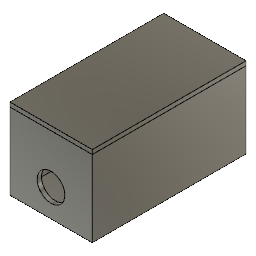
pedal-input (Autodesk Fusion 360 design; units mm, degrees)
Autodesk Fusion 360 part; units mm, degrees
sketch "Sketch1" plane through (0, 0, 0) normal (0, 1, 0) x (1, 0, 0) in component "Case"
  circle A0 centre (0, 0) radius 6.15
  dimension "d9" = 12.3
  constraint coincident A0.centre origin
  measures "d9" diameter of A0
extrude "Extrude2" add sketch "Sketch1" along normal blind 40.4 makes body 1 in component "Case"
sketch "Sketch2" plane through (0, 0, 0) normal (0, -1, 0) x (1, 0, 0) in component "Case"
  circle A0 centre (0, 0) radius 6.15
  circle A1 centre (0, 0) radius 4.85
  dimension "d12" = 9.7
  constraint coincident A0.centre A1.centre
  measures "d12" diameter of A1
extrude "Extrude3" add sketch "Sketch2" along normal blind 2.7 contours A1 bodies 1 in component "Case"
sketch "Sketch3" plane through (0, -2.7, 0) normal (0, -1, 0) x (1, 0, 0) in component "Case"
  circle A0 centre (0, 0) radius 4.85
  circle A1 centre (0, 0) radius 3.3
  dimension "d15" = 6.6
  constraint coincident A0.centre A1.centre
  measures "d15" diameter of A1
extrude "Extrude4" cut sketch "Sketch3" against normal up to surface (42.1 mm away) contours A1 bodies 1 in component "Case"
sketch "Sketch4" plane through (0, 40.4, 0) normal (0, 1, 0) x (-1, 0, 0) in component "Case"
  circle A0 centre (0, 0) radius 6.15
  line L0 (0, 0) -> (2.1, 0)
  line L1 (0, 0) -> (-2.1, 0)
  line L2 (-1.95, 1.525) -> (-2.25, 1.525)
  line L3 (-2.25, 1.525) -> (-2.25, -1.525)
  line L4 (-2.25, -1.525) -> (-1.95, -1.525)
  line L5 (-1.95, -1.525) -> (-1.95, 1.525)
  line L6 (-1.95, 1.525) -> (-2.25, -1.525) construction
  line L7 (-2.25, 1.525) -> (-1.95, -1.525) construction
  line L8 (2.25, 1.525) -> (1.95, 1.525)
  line L9 (1.95, 1.525) -> (1.95, -1.525)
  line L10 (1.95, -1.525) -> (2.25, -1.525)
  line L11 (2.25, -1.525) -> (2.25, 1.525)
  line L12 (2.25, 1.525) -> (1.95, -1.525) construction
  line L13 (1.95, 1.525) -> (2.25, -1.525) construction
  point P0 (-2.1, 0)
  point P1 (2.1, 0)
  dimension "d19" = 2.1
  dimension "d20" = 2.1
  dimension "d21" = 0.3
  dimension "d22" = 3.05
  dimension "d25" = 0.3
  dimension "d26" = 3.05
  constraint coincident A0.centre L0.start
  constraint horizontal L0
  constraint parallel L0 L1
  constraint horizontal L2
  constraint perpendicular L2 L3
  constraint parallel L2 L4
  constraint parallel L3 L5
  constraint coincident L6 P0
  constraint coincident L7 P0
  constraint coincident P0 L1.end
  constraint horizontal L8
  constraint perpendicular L8 L9
  constraint parallel L8 L10
  constraint parallel L9 L11
  constraint coincident L12 P1
  constraint coincident L13 P1
  constraint coincident P1 L0.end
  measures "d19" distance of A0.centre P1
  measures "d20" distance of A0.centre P0
  measures "d21" distance of L3.end L4.end
  measures "d22" distance of L2.end L3.end
  measures "d25" distance of L9.end L10.end
  measures "d26" distance of L8.end L9.end
extrude "Extrude5" add sketch "Sketch4" along normal blind 4 contours L2 L3 L4 L5 | L8 L9 L10 L11 bodies 1 in component "Case"
sketch "Sketch5" plane through (0, 0, 0) normal (0, -1, 0) x (1, 0, 0) in component "Case"
  circle A0 centre (0, 0) radius 4.85
  circle A1 centre (0, 0) radius 6.15
  line L0 (12.95, 8.15) -> (-12.95, 8.15)
  line L1 (-12.95, 8.15) -> (-12.95, -8.15)
  line L2 (-12.95, -8.15) -> (12.95, -8.15)
  line L3 (12.95, -8.15) -> (12.95, 8.15)
  line L4 (12.95, 8.15) -> (-12.95, -8.15) construction
  line L5 (-12.95, 8.15) -> (12.95, -8.15) construction
  line L6 (-12.95, 8.15) -> (12.95, 8.15)
  line L7 (12.95, 8.15) -> (12.95, 17.15)
  line L8 (12.95, 17.15) -> (-12.95, 17.15)
  line L9 (-12.95, 17.15) -> (-12.95, 8.15)
  line L10 (14.45, 6.65) -> (14.45, 18.65)
  line L11 (14.45, 18.65) -> (-14.45, 18.65)
  line L12 (-14.45, 18.65) -> (-14.45, 6.65)
  line L13 (-14.45, 6.65) -> (14.45, 6.65)
  line L14 (-14.45, 9.65) -> (-14.45, -9.65)
  line L15 (-14.45, -9.65) -> (14.45, -9.65)
  line L16 (14.45, -9.65) -> (14.45, 9.65)
  line L17 (14.45, 9.65) -> (-14.45, 9.65)
  dimension "d35" = 25.9
  dimension "d36" = 16.3
  dimension "d37" = 25.9
  dimension "d38" = 9
  dimension "d41" = 1.5
  dimension "d42" = 1.5
  constraint horizontal L0
  constraint perpendicular L0 L1
  constraint parallel L0 L2
  constraint parallel L1 L3
  constraint coincident L4 A0.centre
  constraint coincident L5 A0.centre
  constraint coincident A0.centre A1.centre
  constraint horizontal L6
  constraint vertical L7
  constraint horizontal L8
  constraint vertical L9
  measures "d35" distance of L1.end L2.end
  measures "d36" distance of L0.end L1.end
  measures "d37" distance of L0.end L0.start
  measures "d38" distance of L0.end L8.end
extrude "Extrude6" add sketch "Sketch5" along normal blind 1.5 separate body contours A1 | L0 L1 L3 L6 L13 | L3 L7 L10 L13 L16 L17 | L0 L6 L7 L9 L17 | L1 L9 L12 L13 L14 L17 | L1 L2 L3 L13 L14 L15 L16 | L1 L2 L3 L13 | L7 L8 L9 L17 | L7 L8 L9 L10 L11 L12 L17 makes body 2 in component "Case"
sketch "Sketch6" plane through (0, 0, 0) normal (0, 1, 0) x (-1, 0, 0) in component "Case"
  line L0 (-14.45, 18.65) -> (-14.45, -9.65)
  line L1 (-14.45, -9.65) -> (14.45, -9.65)
  line L2 (14.45, -9.65) -> (14.45, 18.65)
  line L3 (14.45, 18.65) -> (-14.45, 18.65)
  line L4 (-12.95, -8.15) -> (12.95, -8.15)
  line L5 (12.95, -8.15) -> (12.95, 17.15)
  line L6 (12.95, 17.15) -> (-12.95, 17.15)
  line L7 (-12.95, 17.15) -> (-12.95, -8.15)
  circle A0 centre (0, 0) radius 4.85
extrude "Extrude7" add sketch "Sketch6" along normal blind 51.4 contours L0 L1 L2 L3 bodies 1 2 in component "Case"
sketch "Sketch7" plane through (0, 0, 17.15) normal (0, 0, -1) x (1, 0, 0) in component "Case"
  line L0 (12.95, 0) -> (-12.95, 0)
  line L1 (-12.95, 0) -> (-12.95, -51.4)
  line L2 (-12.95, -51.4) -> (12.95, -51.4)
  line L3 (12.95, -51.4) -> (12.95, 0)
  line L4 (12.95, 0) -> (-12.95, -51.4) construction
  line L5 (12.95, -51.4) -> (-12.95, 0) construction
  line L6 (-5, -30.5) -> (5, -30.5)
  line L7 (5, -30.5) -> (5, -45.5)
  line L8 (5, -45.5) -> (-5, -45.5)
  line L9 (-5, -45.5) -> (-5, -30.5)
  line L10 (-5, -30.5) -> (5, -45.5) construction
  line L11 (5, -30.5) -> (-5, -45.5) construction
  point P0 (0, -38)
  dimension "d54" = 10
  dimension "d55" = 15
  constraint coincident L0.start L3.end
  constraint coincident L1.end L2.start
  constraint coincident L2.end L3.start
  constraint coincident L0.end L1.start
  constraint horizontal L6
  constraint perpendicular L6 L7
  constraint parallel L6 L8
  constraint parallel L7 L9
  constraint coincident L10 P0
  constraint coincident L11 P0
  measures "d54" distance of L7.end L8.end
  measures "d55" distance of L6.end L7.end
extrude "Extrude9" add sketch "Sketch7" along normal blind 4 separate body contours L6 L7 L8 L9 makes body 3 in component "Case"
sketch "Sketch8" plane through (0, 0, 13.15) normal (0, 0, -1) x (1, 0, 0) in component "Case"
  line L0 (-5, -45.5) -> (5, -45.5)
  line L1 (5, -45.5) -> (5, -30.5)
  line L2 (5, -30.5) -> (-5, -30.5)
  line L3 (-5, -30.5) -> (-5, -45.5)
  line L4 (12.95, 0) -> (-12.95, 0)
  line L5 (-12.95, 0) -> (-12.95, -51.4)
  line L6 (-12.95, -51.4) -> (12.95, -51.4)
  line L7 (12.95, -51.4) -> (12.95, 0)
  line L8 (12.95, -51.4) -> (-12.95, -51.4)
  line L9 (-12.95, -51.4) -> (-12.95, -17.05)
  line L10 (-12.95, -17.05) -> (12.95, -17.05)
  line L11 (12.95, -17.05) -> (12.95, -51.4)
  dimension "d58" = 25.9
  dimension "d59" = 34.35
  constraint horizontal L8
  constraint vertical L9
  constraint horizontal L10
  constraint vertical L11
  constraint coincident L6.end L7.start
  measures "d58" distance of L6.end L5.end
  measures "d59" distance of L6.end L10.end
extrude "Extrude10" add sketch "Sketch8" along normal blind 1 contours L0 L1 L2 L3 | L5 L6 L7 L8 L9 L10 L11 bodies 3 in component "Case"
sketch "Sketch9" plane through (0, 0, 12.15) normal (0, 0, -1) x (1, 0, 0) in component "Case"
  line L0 (12.95, -17.05) -> (-12.95, -17.05)
  line L1 (-12.95, -17.05) -> (-12.95, -51.4)
  line L2 (-12.95, -51.4) -> (12.95, -51.4)
  line L3 (12.95, -51.4) -> (12.95, -17.05)
  line L4 (4.15, -46.5756) -> (-4.15, -46.5756)
  line L5 (-4.15, -46.5756) -> (-4.15, -56.2244)
  line L6 (-4.15, -56.2244) -> (4.15, -56.2244)
  line L7 (4.15, -56.2244) -> (4.15, -46.5756)
  line L8 (4.15, -46.5756) -> (-4.15, -56.2244) construction
  line L9 (-4.15, -46.5756) -> (4.15, -56.2244) construction
  point P0 (0, -51.4)
  dimension "d65" = 8.3
  constraint horizontal L4
  constraint perpendicular L4 L5
  constraint parallel L4 L6
  constraint parallel L5 L7
  constraint coincident L8 P0
  constraint coincident L9 P0
  constraint midpoint L2 P0
  measures "d65" distance of L5.end L6.end
extrude "Extrude11" add sketch "Sketch9" along normal blind 2.9 contours L2 L4 L5 L7 bodies 3 in component "Case"
sketch "Sketch10" plane through (0, 0, -8.15) normal (0, 0, 1) x (-1, 0, 0) in component "Case"
  line L0 (12.95, 0) -> (-12.95, 0)
  line L1 (-12.95, 0) -> (-12.95, -51.4)
  line L2 (-12.95, -51.4) -> (12.95, -51.4)
  line L3 (12.95, -51.4) -> (12.95, 0)
  line L4 (-12.95, 0) -> (-12.95, -41.9) construction
  line L5 (-12.95, -41.9) -> (12.95, -41.9)
  line L6 (12.95, -41.9) -> (12.95, -35.9)
  line L7 (12.95, -35.9) -> (-12.95, -35.9)
  line L8 (-12.95, -35.9) -> (-12.95, -41.9)
  dimension "d81" = 41.9
  dimension "d82" = 25.9
  dimension "d83" = 6
  constraint coincident L0.end L1.start
  constraint perpendicular L0 L4
  constraint horizontal L5
  constraint vertical L6
  constraint horizontal L7
  constraint vertical L8
  measures "d81" distance of L0.end L4.end
  measures "d82" distance of L4.end L5.end
  measures "d83" distance of L4.end L7.end
extrude "Extrude16" add sketch "Sketch10" along normal blind 6.625 contours L1 L3 L5 L6 L7 L8 bodies 2 in component "Case"
sketch "Sketch11" plane through (0, 35.9, 0) normal (0, -1, 0) x (1, 0, 0) in component "Case"
  line L0 (-12.95, -8.15) -> (12.95, -8.15)
  line L1 (12.95, -8.15) -> (12.95, -1.525)
  line L2 (-12.95, -1.525) -> (-12.95, -8.15)
  line L3 (12.95, -1.525) -> (-12.95, -1.525)
  circle A0 centre (0, 0) radius 6.15
extrude "Extrude17" cut sketch "Sketch11" against normal blind 4.5 contours L3 A0 picked at (-0.9187, -4.796) bodies 2 in component "Case"
sketch "Sketch12" plane through (12.95, 0, 0) normal (-1, 0, 0) x (0, -1, 0) in component "Case"
  line L0 (-41.9, -8.15) -> (-41.9, -1.525)
  line L1 (-41.9, -1.525) -> (-35.9, -1.525)
  line L2 (0, -8.15) -> (0, 17.15)
  line L3 (0, 17.15) -> (-51.4, 17.15)
  line L4 (-51.4, 17.15) -> (-51.4, -8.15)
  line L5 (-35.9, -8.15) -> (0, -8.15)
  line L6 (-51.4, 12.15) -> (-17.05, 12.15)
  line L7 (-25.6375, 10.65) -> (-42.8125, 10.65)
  line L8 (-42.8125, 10.65) -> (-42.8125, 13.65)
  line L9 (-42.8125, 13.65) -> (-25.6375, 13.65)
  line L10 (-25.6375, 13.65) -> (-25.6375, 10.65)
  line L11 (-25.6375, 10.65) -> (-42.8125, 13.65) construction
  line L12 (-42.8125, 10.65) -> (-25.6375, 13.65) construction
  line L13 (-35.9, -1.525) -> (-35.9, -8.15)
  line L14 (-17.05, 12.15) -> (-15.55, 12.15)
  line L15 (-15.55, 12.15) -> (-15.55, 13.65)
  line L16 (-15.55, 13.65) -> (-17.05, 13.65)
  line L17 (-17.05, 13.65) -> (-17.05, 12.15)
  line L18 (-51.4, -8.15) -> (-41.9, -8.15)
  point P0 (-34.225, 12.15)
  dimension "d94" = 17.175
  dimension "d95" = 3
  dimension "d106" = 1.5
  dimension "d107" = 1.5
  constraint horizontal L7
  constraint perpendicular L7 L8
  constraint parallel L7 L9
  constraint parallel L8 L10
  constraint coincident L11 P0
  constraint coincident L12 P0
  constraint midpoint L6 P0
  constraint horizontal L14
  constraint vertical L15
  constraint horizontal L16
  constraint vertical L17
  constraint coincident L6.end L14.start
  measures "d94" distance of L8.end L9.end
  measures "d95" distance of L7.end L8.end
  measures "d106" distance of L6.end L14.end
  measures "d107" distance of L6.end L16.end
extrude "Extrude22" add sketch "Sketch12" along normal blind 3.7 contours L14 L15 L16 L17 bodies 2 in component "Case"
extrude "Extrude20" add sketch "Sketch12" along normal blind 2.59 contours L6 L7 L8 L10 bodies 2 in component "Case"
sketch "Sketch13" plane through (-12.95, 0, 0) normal (1, 0, 0) x (0, 1, 0) in component "Case"
  line L0 (41.9, -1.525) -> (41.9, -8.15)
  line L1 (41.9, -8.15) -> (51.4, -8.15)
  line L2 (51.4, -8.15) -> (51.4, 17.15)
  line L3 (51.4, 17.15) -> (0, 17.15)
  line L4 (0, 17.15) -> (0, -8.15)
  line L5 (35.9, -1.525) -> (41.9, -1.525)
  line L6 (17.05, 12.15) -> (51.4, 12.15)
  line L7 (42.8125, 10.65) -> (25.6375, 10.65)
  line L8 (25.6375, 10.65) -> (25.6375, 13.65)
  line L9 (25.6375, 13.65) -> (42.8125, 13.65)
  line L10 (42.8125, 13.65) -> (42.8125, 10.65)
  line L11 (42.8125, 10.65) -> (25.6375, 13.65) construction
  line L12 (25.6375, 10.65) -> (42.8125, 13.65) construction
  line L13 (0, -8.15) -> (35.9, -8.15)
  line L14 (35.9, -8.15) -> (35.9, -1.525)
  line L15 (17.05, 12.15) -> (15.55, 12.15)
  line L16 (15.55, 12.15) -> (15.55, 13.65)
  line L17 (15.55, 13.65) -> (17.05, 13.65)
  line L18 (17.05, 13.65) -> (17.05, 12.15)
  point P0 (34.225, 12.15)
  dimension "d98" = 17.175
  dimension "d99" = 3
  dimension "d114" = 1.5
  dimension "d115" = 1.5
  constraint horizontal L7
  constraint perpendicular L7 L8
  constraint parallel L7 L9
  constraint parallel L8 L10
  constraint coincident L11 P0
  constraint coincident L12 P0
  constraint midpoint L6 P0
  constraint horizontal L15
  constraint vertical L16
  constraint horizontal L17
  constraint vertical L18
  constraint coincident L6.start L15.start
  measures "d98" distance of L8.end L9.end
  measures "d99" distance of L7.end L8.end
  measures "d114" distance of L6.start L15.end
  measures "d115" distance of L6.start L17.end
extrude "Extrude23" add sketch "Sketch13" along normal blind 3.7 contours L15 L16 L17 L18 bodies 2 in component "Case"
extrude "Extrude21" add sketch "Sketch13" along normal blind 2.59 contours L6 L7 L8 L10 bodies 2 in component "Case"
sketch "Sketch14" plane through (0, 51.4, 0) normal (0, 1, 0) x (-1, 0, 0) in component "Case"
  line L0 (-12.95, -8.15) -> (-12.95, 17.15)
  line L1 (-12.95, 17.15) -> (12.95, 17.15)
  line L2 (12.95, -8.15) -> (-12.95, -8.15)
  line L3 (14.45, 18.65) -> (-14.45, 18.65)
  line L4 (-14.45, 18.65) -> (-14.45, -9.65)
  line L5 (-14.45, -9.65) -> (14.45, -9.65)
  line L6 (14.45, -9.65) -> (14.45, 18.65)
  line L7 (12.95, 17.15) -> (12.95, -8.15)
extrude "Extrude18" add sketch "Sketch14" along normal blind 1 contours L0 L1 L2 L7 | L3 L4 L5 L6 bodies 2 in component "Case"
sketch "Sketch15" plane through (0, 51.4, 0) normal (0, 1, 0) x (-1, 0, 0) in component "Case"
  line L0 (12.95, 13.15) -> (-12.95, 13.15)
  line L1 (-12.95, 13.15) -> (-12.95, 12.15)
  line L2 (-12.95, 12.15) -> (-4.15, 12.15)
  line L3 (-4.15, 12.15) -> (-4.15, 9.25)
  line L4 (-4.15, 9.25) -> (4.15, 9.25)
  line L5 (4.15, 9.25) -> (4.15, 12.15)
  line L6 (4.15, 12.15) -> (12.95, 12.15)
  line L7 (12.95, 12.15) -> (12.95, 13.15)
  line L8 (-4.15, 12.15) -> (4.15, 12.15)
  dimension "d91" = 8.3
  constraint coincident L2.end L3.start
  constraint coincident L5.end L6.start
  measures "d91" distance of L2.end L5.end
extrude "Extrude19" cut sketch "Sketch15" along normal blind 1 contours L3 L4 L5 L8 bodies 2 in component "Case"
fillet "Fillet2" [suppressed] in component "Case"
split "Split1" by plane through (-12.95, 0, 17.15) normal (0, 0, -1) bodies 2 makes body 4 at (4.8167, 16.4667, -9.65) in component "Case"
component "Case" placed x (1, 0, 0) y (0, 1, 0) z (0, 0, 1) at (0, 0, 0)
hidden bodies 1 3
equation "JackLength = 39.4 mm + 1 mm" comment "Length of the jack without contacts or lip"
equation "JackDiameter = 11.3 mm + 1 mm" comment "Diameter of the jack"
equation "JackLipLength = 2.7 mm" comment "Length/height of the lip in the front of the jack"
equation "JackLipDiameter = 8.7 mm + 1 mm" comment "Diameter of the lip in the front of the jack"
equation "d9 = JackDiameter"
equation "d10 = JackLength"
equation "d12 = JackLipDiameter"
equation "d13 = JackLipLength"
equation "JackContactSpacing = 4.2 mm" comment "Space between the two contacts on the back of the jack"
equation "d19 = JackContactSpacing / 2"
equation "d20 = JackContactSpacing / 2"
equation "d21 = JackContactThickness"
equation "d22 = JackContactHeight"
equation "JackContactThickness = 0.3 mm" comment "Thickness of the contacts on the back of the jack"
equation "JackContactHeight = 2.8 mm + 0.25 mm" comment "Height of the contacts on the back of the jack"
equation "d25 = JackContactThickness"
equation "d26 = JackContactHeight"
equation "JackContactLength = 4 mm" comment "Length of the contact on the back of the jack"
equation "d28 = JackContactLength"
equation "ChipWidth = 25.4 mm + 0.5 mm" comment "Width of the Chip"
equation "ChipLength = 34.1 mm + 0.25 mm" comment "Length of the Chip"
equation "ChipThickness = 1 mm" comment "Chip PCB thickness"
equation "ChipBellyThickness = 3 mm + 1 mm" comment "Thickness/height of the \"belly\" of the chip"
equation "JackSpacing = 2 mm" comment "Space above and below jack"
equation "d35 = ChipWidth"
equation "d36 = 2 * ( JackDiameter / 2 + JackSpacing )"
equation "d37 = ChipWidth"
equation "d38 = ChipSpacing * 2 + ChipBellyThickness + ChipThickness"
equation "ChipSpacing = 2 mm" comment "Spacing under chip"
equation "WallThickness = 1.5 mm" comment "Thickness of all walls"
equation "d41 = WallThickness"
equation "d42 = WallThickness"
equation "d43 = WallThickness"
equation "d45 = -WallThickness"
equation "JackBackSpacing = 5 mm" comment "Spacing behind the contacts of the jack"
equation "d47 = JackLength + JackContactLength + ChipSpacing + JackBackSpacing"
equation "ChipUSBThickness = 2.4 mm + 0.5 mm" comment "Thickness/height of the USB connector"
equation "d56 = ChipBellyThickness"
equation "d58 = ChipWidth"
equation "d59 = ChipLength"
equation "d60 = ChipThickness"
equation "d62 = ChipUSBThickness"
equation "ChipUSBWidth = 7.8 mm + 0.5 mm" comment "Width of USB connector"
equation "d65 = ChipUSBWidth"
equation "d81 = JackLength + WallThickness"
equation "d82 = ChipWidth"
equation "d83 = WallThickness * 4"
equation "d84 = JackSpacing + JackDiameter / 2 - JackContactHeight / 2"
equation "CaseBackWallThickness = 1 mm" comment "Thickness of back wall, needs to be smaller for USB cable to reach through"
equation "d89 = CaseBackWallThickness"
equation "d91 = ChipUSBWidth"
equation "d92 = CaseBackWallThickness"
equation "d94 = ChipLength / 2"
equation "d95 = WallThickness * 2"
equation "d96 = ChipWidth / 10"
equation "d98 = ChipLength / 2"
equation "d99 = WallThickness * 2"
equation "d100 = ChipWidth / 10"
equation "d105 = WallThickness"
equation "d106 = WallThickness"
equation "d107 = ChipThickness * 1.5"
equation "d108 = ChipWidth / 7"
equation "d112 = ChipWidth / 7"
equation "d114 = WallThickness"
equation "d115 = ChipThickness * 1.5"
named bodies: "Jack", "Cover", "Chip", "Case"
